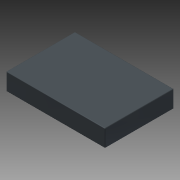
# Autodesk Inventor part: HDD3.5
Saved by Autodesk Inventor 2015 (Build 190159000, 159)
## iProperties
Created: 2016-03-23
Part Number: HDD3.5
Material: Generic
Document SubType Name: Modeling
Designer: Noah
Density: 1 g/cm^3
Appearance: Default
Author: Noah
Autodesk Inventor part; units mm, degrees
ref_plane "YZ Plane" through (0, 0, 0) normal (1, 0, 0) x (0, 1, 0)
ref_plane "XZ Plane" through (0, 0, 0) normal (0, 1, 0) x (-1, 0, 0)
ref_plane "XY Plane" through (0, 0, 0) normal (0, 0, 1) x (1, 0, 0)
sketch "Sketch1" plane through (0, 0, 0) normal (0, 0, 1) x (1, 0, 0)
  line L0 (-73, 50.8) -> (73, 50.8)
  line L1 (73, 50.8) -> (73, -50.8)
  line L2 (73, -50.8) -> (-73, -50.8)
  line L3 (-73, -50.8) -> (-73, 50.8)
  point P0 (0, 0)
  dimension "d0" = 146
  dimension "d1" = 101.6
  dimension "d2" = 50.8
  dimension "d3" = 73
  constraints: 8 end point, 2 parallel, 1 horizontal, 1 perpendicular
  measures "d0" distance of L1.end L2.end
  measures "d1" distance of L0.end L1.end
  measures "d2" distance from line of L0 point (0, 0)
  measures "d3" distance from line of point (0, 0) L1
extrude "Extrusion1" add sketch "Sketch1" along normal blind 25.4
fillet "Fillet1" radius 1 12 edges at (0, 50.8, 25.4) (0, 50.8, 0) (0, -50.8, 25.4) (73, 0, 0) (-73, 0, 0) (73, 50.8, 12.7) (73, -50.8, 12.7) (73, 0, 25.4) (-73, 0, 25.4) (-73, 50.8, 12.7) (-73, -50.8, 12.7) (0, -50.8, 0)
body "Solid1"
